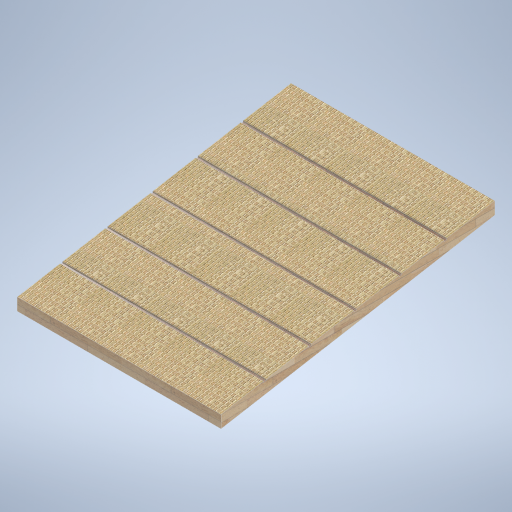
# Autodesk Inventor part: eave_panel_02
Saved by Autodesk Inventor 2024.2 (Build 282272000, 272)
## iProperties
Created: 2024-05-23
Part Number: eave_panel_02
Material: Wood (Maple)
Document SubType Name: Modeling
Designer: LOSTER_1
Density: 0.67 g/cm^3
Appearance: Natural Maple - Glossy Dark Tint
Author: LOSTER_1
Autodesk Inventor part; units mm, degrees
ref_plane "YZ Plane" through (0, 0, 0) normal (1, 0, 0) x (0, 1, 0)
ref_plane "XZ Plane" through (0, 0, 0) normal (0, 1, 0) x (-1, 0, 0)
sketch "Sketch1" plane through (0, 0, 0) normal (0, 0, 1) x (1, 0, 0)
  line L0 (-822, 50) -> (822, 50)
  line L1 (822, 50) -> (822, -50)
  line L2 (822, -50) -> (-822, -50)
  line L3 (-822, -50) -> (-822, 50)
  line L4 (-822, 50) -> (822, -50) construction
  line L5 (822, 50) -> (-822, -50) construction
  point P0 (0, 0)
  dimension "d0" = 1644
  dimension "d1" = 100
  constraints: 12 end point, 2 midpoint, 2 parallel, 1 horizontal, 1 perpendicular
  measures "d0" distance of L1.end L2.end
  measures "d1" distance of L0.end L1.end
ref_plane "Work Plane2" through (0, 0, 2209) normal (0, 0, 1) x (1, 0, 0)
ref_plane "Work Plane1" through (0, 0, 0) normal (0, 0, 1) x (1, 0, 0)
sketch "Sketch2" plane through (0, 0, 2209) normal (0, 0, 1) x (1, 0, 0)
  line L0 (-822, -50) -> (-822, 50) projected
  line L1 (822, 50) -> (822, -50) projected
  point P0 (0, 0)
ref_plane "Work Plane3" through (-822, -50, 0) normal (1, 0, 0) x (0, 1, 0)
sketch "Sketch3" plane through (-822, -50, 0) normal (1, 0, 0) x (0, 1, 0)
  line L0 (0, 0) -> (100, 0) projected
  line L1 (0, 2209) -> (100, 2209) projected
  line L2 (100, 0) -> (-289.5063, 2209)
  line L3 (100, 0) -> (2343.0774, 0) construction
  line L4 (0, 0) -> (-389.5063, 2209)
  line L5 (0, 0) -> (2243.0774, 0) construction
  line L6 (-389.5063, 2209) -> (0, 2209)
  point P0 (50, 0)
  dimension "d4" = 100
  dimension "d5" = 100
  constraints: 10 end point, 3 horizontal, 2 equal length
  measures "d4" angle of L3 L2
  measures "d5" angle of L5 L4
sketch "Sketch4" plane through (0, 0, 2209) normal (0, 0, 1) x (1, 0, 0)
  line L0 (-822, -439.5063) -> (-822, -50) projected
  line L1 (-822, -339.5063) -> (822, -339.5063)
  line L2 (822, -339.5063) -> (822, -439.5063)
  line L3 (822, -439.5063) -> (-822, -439.5063)
  line L4 (-822, -439.5063) -> (-822, -339.5063)
  point P0 (0, 0)
  dimension "d6" = 1644
  constraints: 8 end point, 2 parallel, 1 horizontal, 1 perpendicular
  measures "d6" distance of L2.end L3.end
loft "Loft1" add profiles "Sketch4", "Sketch1"
sketch "Sketch5" plane through (822, -439.5063, 2209) normal (1, 0, 0) x (0, 0, -1)
  line L0 (0, 100) -> (0, 0) projected
  line L1 (0, 0) -> (2209, 389.5063) projected
  line L2 (2209, 489.5063) -> (2209, 389.5063) projected
  line L3 (0, 100) -> (2209, 489.5063) projected
  line L4 (0, 100) -> (344.6827, 160.7769)
  line L5 (0, 100) -> (2209, 489.5063) projected
  line L6 (344.6827, 160.7769) -> (344.6827, 150.9175)
  line L7 (344.6827, 150.9175) -> (364.3393, 154.3835)
  line L8 (364.3393, 154.3835) -> (364.3393, 164.2429)
  line L9 (364.3393, 164.2429) -> (709.022, 225.0197)
  line L10 (709.022, 225.0197) -> (709.022, 215.1603)
  line L11 (709.022, 215.1603) -> (729.0699, 218.6953)
  line L12 (729.0699, 218.6953) -> (729.0699, 228.5547)
  line L13 (729.0699, 228.5547) -> (1073.7526, 289.3316)
  line L14 (1073.7526, 289.3316) -> (1073.7526, 279.4722)
  line L15 (1073.7526, 279.4722) -> (1092.9888, 282.864)
  line L16 (1092.9888, 282.864) -> (1092.9888, 292.7234)
  line L17 (1092.9888, 292.7234) -> (1437.6715, 353.5003)
  line L18 (1437.6715, 353.5003) -> (1437.6715, 343.6409)
  line L19 (1437.6715, 343.6409) -> (1457.7333, 347.1783)
  line L20 (1457.7333, 347.1783) -> (1457.7333, 357.0377)
  line L21 (1457.7333, 357.0377) -> (1802.416, 417.8146)
  line L22 (1802.416, 417.8146) -> (1802.416, 407.9552)
  line L23 (1802.416, 407.9552) -> (1822.281, 411.4579)
  line L24 (1822.281, 411.4579) -> (1822.281, 421.3173)
  line L25 (1822.281, 421.3173) -> (2209, 489.5063)
  line L26 (1822.281, 421.3173) -> (344.6827, 160.7769)
  point P0 (2209, 439.5063)
  point P1 (709.022, 225.0197)
  point P2 (364.3393, 164.2429)
  point P3 (344.6827, 160.7769)
  dimension "d11" = 350
  dimension "d12" = 350
  dimension "d13" = 350
  dimension "d14" = 350
  dimension "d15" = 350
  constraints: 44 end point, 9 parallel, 8 point on line, 1 collinear, 1 vertical, 11 other
  measures "d11" distance of L0.start L4.end
  measures "d12" distance of L8.end L9.end
  measures "d13" distance of L12.end L13.end
  measures "d14" distance of L16.end L17.end
  measures "d15" distance of L20.end L21.end
extrude "Extrusion1" cut sketch "Sketch5" against normal through all contours L3 L8 L7 L6 | L3 L12 L11 L10 | L24 L23 L22 L3 | L3 L16 L15 L14 | L20 L19 L18 L3
body "Solid1"
